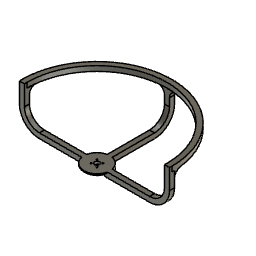
symmetrical_propeller_guard v3 (Autodesk Fusion 360 design; units mm, degrees)
Autodesk Fusion 360 part; units mm, degrees
sketch "Sketch1" plane through (0, 0, 0) normal (0, 0, 1) x (1, 0, 0)
  circle A0 centre (0, 0) radius 26
  dimension "d1" = 52
  constraint coincident A0.centre origin
  measures "d1" diameter of A0
extrude "Extrude1" add sketch "Sketch1" along normal blind 10
sketch "Sketch2" plane through (0, 0, 0) normal (0, 1, 0) x (1, 0, 0)
  line L0 (0, 0) -> (110, 0)
  arc A0 (150, -40) -> (110, 0) centre (110, -40) ccw
  line L1 (150, -40) -> (150, -70)
  line L2 (150, -70) -> (140, -70)
  arc A1 (140, -40) -> (110, -10) centre (110, -40) ccw
  line L3 (140, -70) -> (140, -40)
  line L4 (110, -10) -> (0, -10)
  line L5 (0, -10) -> (0, 0)
  dimension "d4" = 110
  dimension "d5" = 110
  dimension "d6" = 10
  dimension "d7" = 30
  dimension "d8" = 40
  dimension "d9" = 10
  constraint coincident L0.start L5.end
  constraint horizontal L0
  constraint tangent A0 L1
  constraint vertical L1
  constraint perpendicular L1 L2
  constraint coincident A0.centre A1.centre
  constraint tangent A1 L3
  constraint tangent A1 L4
  constraint perpendicular L3 L4
  constraint perpendicular L0 L5
  measures "d4" distance of L0.start L0.end
  measures "d5" distance of A1.end L4.end
  measures "d6" distance of L4.end L0.start
  measures "d7" radius of A1
  measures "d8" radius of A0
  measures "d9" distance of L1.end L2.end
extrude "Extrude2" add sketch "Sketch2" along normal mid plane 10
pattern_circular "C-Pattern1" count 3 over 180 about axis through (0, 0, 1.75) along (0, 0, 1) of "Extrude2"
sketch "Sketch3" plane through (0, 0, 70) normal (0, 0, 1) x (-1, 0, 0)
  line L0 (-150, 5) -> (-150, -5)
  line L1 (-150, -5) -> (-140, -5)
  line L2 (-140, -5) -> (-140, 5)
  line L3 (-140, 5) -> (-150, 5)
  arc A0 (-140, 0) -> (140, 0) centre (0, 0) ccw
  arc A1 (-150, 0) -> (150, 0) centre (0, 0) ccw
  line L4 (150, 0) -> (150, 5)
  line L5 (150, 5) -> (140, 5)
  line L6 (140, 5) -> (140, 0)
  line L7 (-150, 0) -> (-150, 5)
  line L8 (-140, 5) -> (-140, 0)
  constraint tangent L2 A0
  constraint tangent L0 A1
  constraint tangent A1 L4
  constraint vertical L4
  constraint perpendicular L4 L5
  constraint tangent A0 L6
  constraint coincident L0.start L3.end
  constraint tangent A1 L7
  constraint coincident L2.end L3.start
  constraint tangent A0 L8
extrude "Extrude3" add sketch "Sketch3" along normal blind 10 contours L0 L1 L2 L3 A1 L7 L8 | L1 L2 A0 A1 L4 L5 L6
fillet "Fillet1" chord length 20 4 edges at (144.9583, 5, 70) (5, 144.9583, 70) (-144.9583, 5, 70) (-5, 144.9583, 70)
sketch "Sketch4" plane through (0, 0, 0) normal (0, 0, -1) x (1, 0, 0)
  arc A0 (-25.5147, -5) -> (-5, -25.5147) centre (0, 0) ccw
  line L0 (-5, -25.5147) -> (-5, -110)
  line L1 (-5, -110) -> (5, -110)
  line L2 (5, -110) -> (5, -25.5147)
  arc A1 (5, -25.5147) -> (25.5147, -5) centre (0, 0) ccw
  line L3 (25.5147, -5) -> (110, -5)
  line L4 (110, -5) -> (110, 5)
  line L5 (110, 5) -> (25.5147, 5)
  arc A2 (25.5147, 5) -> (-25.5147, 5) centre (0, 0) ccw
  line L6 (-25.5147, 5) -> (-110, 5)
  line L7 (-110, 5) -> (-110, -5)
  line L8 (-110, -5) -> (-25.5147, -5)
  circle A3 centre (0, 0) radius 20.5
  line L9 (-30, 30) -> (30, 30)
  line L10 (30, 30) -> (30, 5)
  line L11 (30, 5) -> (-30, 5)
  line L12 (-30, 5) -> (-30, 30)
  dimension "d39" = 41
  constraint concentric A0 A3
  constraint horizontal L9
  constraint vertical L10
  constraint horizontal L11
  constraint vertical L12
  constraint coincident L5 L10.end
  measures "d39" diameter of A3
extrude "Extrude5" cut sketch "Sketch4" against normal blind 5 contours L5 A2 L6 L9 L10 L11 L12 | A2 A3 L11 | A3 L11 | A3 L11
chamfer "Chamfer1" distance 3 angle 45 1 edges at (0, -26, 5)
sketch "Sketch5" plane through (0, 0, 10) normal (0, 0, 1) x (-1, 0, 0)
  arc A0 (25.5147, 5) -> (-25.5147, 5) centre (0, 0) ccw
  line L0 (-25.5147, 5) -> (-110, 5)
  line L1 (-110, 5) -> (-110, -5)
  line L2 (-110, -5) -> (-25.5147, -5)
  arc A1 (-25.5147, -5) -> (-5, -25.5147) centre (0, 0) ccw
  line L3 (-5, -25.5147) -> (-5, -110)
  line L4 (-5, -110) -> (5, -110)
  line L5 (5, -110) -> (5, -25.5147)
  arc A2 (5, -25.5147) -> (25.5147, -5) centre (0, 0) ccw
  line L6 (25.5147, -5) -> (110, -5)
  line L7 (110, -5) -> (110, 5)
  line L8 (110, 5) -> (25.5147, 5)
  circle A3 centre (0, 0) radius 5
  circle A4 centre (-5.6569, -5.6569) radius 1.5
  circle A5 centre (6.7175, -6.7175) radius 1.5
  circle A6 centre (5.6569, 5.6569) radius 1.5
  circle A7 centre (-6.7175, 6.7175) radius 1.5
  dimension "d26" = 10
  dimension "d27" = 3
  dimension "d28" = 3
  dimension "d29" = 8
  dimension "d30" = 9.5
  dimension "d31" = 6.7175
  dimension "d32" = 5.6569
  dimension "d34" = 360
  constraint coincident A0.centre A1.centre
  measures "d26" diameter of A3
  measures "d27" diameter of A4
  measures "d28" diameter of A5
  measures "d29" distance of A0.centre A4.centre
  measures "d30" distance of A0.centre A5.centre
  measures "d31" horizontal distance of A0.centre A5.centre
  measures "d32" horizontal distance of A0.centre A4.centre
extrude "Extrude6" cut sketch "Sketch5" against normal blind 5 contours A3 | A4 | A5 | A6 | A7
move_body "Move1" [suppressed]
mirror "Mirror1" [suppressed]
